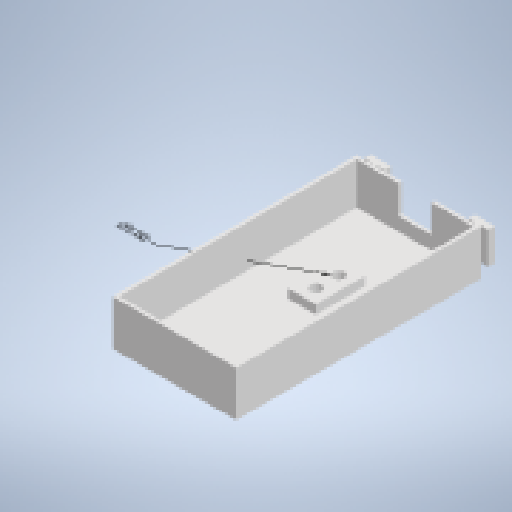
# Autodesk Inventor part: Soporte_Cuenco
Saved by Autodesk Inventor 2024 (Build 280153000, 153)
## iProperties
Created: 2024-07-17
Part Number: Soporte_Cuenco
Material: Genérico
Document SubType Name: Modeling
Designer: sergi
Density: 1 g/cm^3
Appearance: Valor por defecto
Author: sergi
Autodesk Inventor part; units mm, degrees
ref_plane "YZ Plane" through (0, 0, 0) normal (1, 0, 0) x (0, 1, 0)
ref_plane "XZ Plane" through (0, 0, 0) normal (0, 1, 0) x (-1, 0, 0)
ref_plane "XY Plane" through (0, 0, 0) normal (0, 0, 1) x (1, 0, 0)
sketch "Boceto1" plane through (0, 0, 0) normal (0, 0, 1) x (1, 0, 0)
  line L0 (-21.643, 32.4807) -> (-21.643, 43.3467) projected
  line L1 (-21.643, 43.3467) -> (-18.643, 43.3467) projected
  line L2 (-18.643, 43.3467) -> (-18.643, 34.2127) projected
  line L3 (-18.643, 34.2127) -> (-9.9759, 39.2167) projected
  line L4 (-9.9759, 39.2167) -> (9.7759, 39.2167) projected
  line L5 (9.7759, 39.2167) -> (18.443, 34.2127) projected
  line L6 (18.443, 34.2127) -> (18.443, 43.3467) projected
  line L7 (18.443, 43.3467) -> (21.443, 43.3467) projected
  line L8 (21.443, 43.3467) -> (21.443, 32.4807) projected
  line L9 (21.443, 32.4807) -> (29.5244, 27.8149) projected
  ellipse E0 centre (28.1102, 26.9984) end of major axis (26.1102, 26.9984) minor radius 1.1547 (30.1102, 26.9984) -> (29.5244, 27.8149) ccw projected
  line L10 (30.1102, 26.9984) -> (30.1102, 16.9984) projected
  line L11 (30.1102, 16.9984) -> (-30.3102, 16.9984) projected
  line L12 (-30.3102, 16.9984) -> (-30.3102, 26.9984) projected
  ellipse E1 centre (-28.3102, 26.9984) end of major axis (-30.3102, 26.9984) minor radius 1.1547 (-29.7244, 27.8149) -> (-30.3102, 26.9984) ccw projected
  line L13 (-29.7244, 27.8149) -> (-21.643, 32.4807) projected
  circle A0 centre (-50.1, -10) radius 1.5 projected
  circle A1 centre (49.9, -10) radius 1.5 projected
  circle A2 centre (49.9, 113) radius 1.5 projected
  circle A3 centre (-50.1, 113) radius 1.5 projected
  circle A4 centre (-50.1, -110) radius 1.75 projected
  circle A5 centre (49.9, -110) radius 1.75 projected
  line L14 (-22.1, 125) -> (-22.1, 110) projected
  line L15 (-22.1, 110) -> (-25.1, 110) projected
  line L16 (-25.1, 110) -> (-25.1, 125) projected
  line L17 (-25.1, 125) -> (-103.1, 125) projected
  line L18 (-103.1, 125) -> (-103.1, 100) projected
  line L19 (-103.1, 100) -> (-100.1, 100) projected
  line L20 (-100.1, 100) -> (-100.1, 75) projected
  line L21 (-100.1, 75) -> (-103.1, 75) projected
  line L22 (-103.1, 75) -> (-103.1, 50) projected
  line L23 (-103.1, 50) -> (-100.1, 50) projected
  line L24 (-100.1, 50) -> (-100.1, 25) projected
  line L25 (-100.1, 25) -> (-103.1, 25) projected
  line L26 (-103.1, 25) -> (-103.1, 0) projected
  line L27 (-103.1, 0) -> (-100.1, 0) projected
  line L28 (-100.1, 0) -> (-100.1, -25) projected
  line L29 (-100.1, -25) -> (-103.1, -25) projected
  line L30 (-103.1, -25) -> (-103.1, -50) projected
  line L31 (-103.1, -50) -> (-100.1, -50) projected
  line L32 (-100.1, -50) -> (-100.1, -75) projected
  line L33 (-100.1, -75) -> (-103.1, -75) projected
  line L34 (-103.1, -75) -> (-103.1, -100) projected
  line L35 (-103.1, -100) -> (-100.1, -100) projected
  line L36 (-100.1, -100) -> (-100.1, -125) projected
  line L37 (-100.1, -125) -> (102.9, -125) projected
  line L38 (102.9, -125) -> (102.9, -100) projected
  line L39 (102.9, -100) -> (99.9, -100) projected
  line L40 (99.9, -100) -> (99.9, -75) projected
  line L41 (99.9, -75) -> (102.9, -75) projected
  line L42 (102.9, -75) -> (102.9, -50) projected
  line L43 (102.9, -50) -> (99.9, -50) projected
  line L44 (99.9, -50) -> (99.9, -25) projected
  line L45 (99.9, -25) -> (102.9, -25) projected
  line L46 (102.9, -25) -> (102.9, 0) projected
  line L47 (102.9, 0) -> (99.9, 0) projected
  line L48 (99.9, 0) -> (99.9, 25) projected
  line L49 (99.9, 25) -> (102.9, 25) projected
  line L50 (102.9, 25) -> (102.9, 50) projected
  line L51 (102.9, 50) -> (99.9, 50) projected
  line L52 (99.9, 50) -> (99.9, 75) projected
  line L53 (99.9, 75) -> (102.9, 75) projected
  line L54 (102.9, 75) -> (102.9, 100) projected
  line L55 (102.9, 100) -> (99.9, 100) projected
  line L56 (99.9, 100) -> (99.9, 125) projected
  line L57 (99.9, 125) -> (24.9, 125) projected
  line L58 (24.9, 125) -> (24.9, 110) projected
  line L59 (24.9, 110) -> (21.9, 110) projected
  line L60 (21.9, 110) -> (21.9, 125) projected
  line L61 (24.9, 125) -> (21.9, 125)
  line L62 (22.15, 125.25) -> (22.15, 110.25)
  line L63 (22.15, 110.25) -> (24.65, 110.25)
  line L64 (24.65, 110.25) -> (24.65, 125.25)
  line L65 (24.65, 125.25) -> (100.15, 125.25)
  line L66 (100.15, 125.25) -> (100.15, 100.25)
  line L67 (100.15, 100.25) -> (103.15, 100.25)
  line L68 (103.15, 100.25) -> (103.15, 74.75)
  line L69 (103.15, 74.75) -> (100.15, 74.75)
  line L70 (100.15, 74.75) -> (100.15, 50.25)
  line L71 (100.15, 50.25) -> (103.15, 50.25)
  line L72 (103.15, 50.25) -> (103.15, 24.75)
  line L73 (103.15, 24.75) -> (100.15, 24.75)
  line L74 (100.15, 24.75) -> (100.15, 0.25)
  line L75 (100.15, 0.25) -> (103.15, 0.25)
  line L76 (103.15, 0.25) -> (103.15, -25.25)
  line L77 (103.15, -25.25) -> (100.15, -25.25)
  line L78 (100.15, -25.25) -> (100.15, -49.75)
  line L79 (100.15, -49.75) -> (103.15, -49.75)
  line L80 (103.15, -49.75) -> (103.15, -75.25)
  line L81 (103.15, -75.25) -> (100.15, -75.25)
  line L82 (100.15, -75.25) -> (100.15, -99.75)
  line L83 (100.15, -99.75) -> (103.15, -99.75)
  line L84 (103.15, -99.75) -> (103.15, -125.25)
  line L85 (103.15, -125.25) -> (-100.35, -125.25)
  line L86 (-100.35, -125.25) -> (-100.35, -100.25)
  line L87 (-100.35, -100.25) -> (-103.35, -100.25)
  line L88 (-103.35, -100.25) -> (-103.35, -74.75)
  line L89 (-103.35, -74.75) -> (-100.35, -74.75)
  line L90 (-100.35, -74.75) -> (-100.35, -50.25)
  line L91 (-100.35, -50.25) -> (-103.35, -50.25)
  line L92 (-103.35, -50.25) -> (-103.35, -24.75)
  line L93 (-103.35, -24.75) -> (-100.35, -24.75)
  line L94 (-100.35, -24.75) -> (-100.35, -0.25)
  line L95 (-100.35, -0.25) -> (-103.35, -0.25)
  line L96 (-103.35, -0.25) -> (-103.35, 25.25)
  line L97 (-103.35, 25.25) -> (-100.35, 25.25)
  line L98 (-100.35, 25.25) -> (-100.35, 49.75)
  line L99 (-100.35, 49.75) -> (-103.35, 49.75)
  line L100 (-103.35, 49.75) -> (-103.35, 75.25)
  line L101 (-103.35, 75.25) -> (-100.35, 75.25)
  line L102 (-100.35, 75.25) -> (-100.35, 99.75)
  line L103 (-100.35, 99.75) -> (-103.35, 99.75)
  line L104 (-103.35, 99.75) -> (-103.35, 125.25)
  line L105 (-103.35, 125.25) -> (-24.85, 125.25)
  line L106 (-24.85, 125.25) -> (-24.85, 110.25)
  line L107 (-24.85, 110.25) -> (-22.35, 110.25)
  line L108 (-22.35, 110.25) -> (-22.35, 125.25)
  line L109 (-22.35, 125.25) -> (22.15, 125.25)
  line L110 (24.9418, 124.75) -> (21.9418, 124.75)
  line L111 (-22.1, 125) -> (-25.1, 125)
  line L112 (-22.0582, 124.75) -> (-25.0582, 124.75)
  line L113 (7.4, 125) -> (7.4, 115) projected
  line L114 (7.4, 115) -> (-7.6, 115) projected
  line L115 (-7.6, 115) -> (-7.6, 125) projected
  line L116 (-7.6, 125) -> (-22.1, 125) projected
  line L117 (21.9, 125) -> (7.4, 125) projected
  point P0 (0, 0)
  point P1 (-22.35, 124.75)
  point P2 (-24.85, 124.75)
  point P3 (24.65, 124.75)
  point P4 (22.15, 124.75)
  dimension "d0" = 0.25
  dimension "d1" = 0.25
  dimension "d2" = 0.25
  constraints: 104 end point, 2 horizontal, 2 parallel, 48 other
  measures "d0" distance between parallel lines of L60 L62
  measures "d1" distance between parallel lines of L61 L110
  measures "d2" distance between parallel lines of L111 L112
extrude "Extrusión1" add sketch "Boceto1" against normal blind 3.5 contours L108 L107 L106 L112 | L110 L64 L63 L62
sketch "Boceto2" plane through (0, 0, -3.5) normal (0, 0, -1) x (-1, 0, 0)
  line L0 (22.35, 124.75) -> (22.35, 110.25) projected
  line L1 (22.35, 110.25) -> (24.85, 110.25) projected
  line L2 (24.85, 110.25) -> (24.85, 124.75) projected
  line L3 (24.85, 124.75) -> (22.35, 124.75) projected
  line L4 (-24.65, 124.75) -> (-24.65, 110.25) projected
  line L5 (-24.65, 110.25) -> (-22.15, 110.25) projected
  line L6 (-22.15, 110.25) -> (-22.15, 124.75) projected
  line L7 (-22.15, 124.75) -> (-24.65, 124.75) projected
  circle A0 centre (50.1, -10) radius 1.5 projected
  circle A1 centre (-49.9, -10) radius 1.5 projected
  circle A2 centre (-49.9, 113) radius 1.5 projected
  circle A3 centre (50.1, 113) radius 1.5 projected
  circle A4 centre (50.1, -110) radius 1.75 projected
  circle A5 centre (-49.9, -110) radius 1.75 projected
  line L8 (25.1, 125) -> (25.1, 110) projected
  line L9 (25.1, 110) -> (22.1, 110) projected
  line L10 (22.1, 110) -> (22.1, 125) projected
  line L11 (22.1, 125) -> (7.6, 125) projected
  line L12 (-21.9, 125) -> (-21.9, 110) projected
  line L13 (-21.9, 110) -> (-24.9, 110) projected
  line L14 (-24.9, 110) -> (-24.9, 125) projected
  line L15 (-24.9, 125) -> (-99.9, 125) projected
  line L16 (-99.9, 125) -> (-99.9, 100) projected
  line L17 (-99.9, 100) -> (-102.9, 100) projected
  line L18 (-102.9, 100) -> (-102.9, 75) projected
  line L19 (-102.9, 75) -> (-99.9, 75) projected
  line L20 (-99.9, 75) -> (-99.9, 50) projected
  line L21 (-99.9, 50) -> (-102.9, 50) projected
  line L22 (-102.9, 50) -> (-102.9, 25) projected
  line L23 (-102.9, 25) -> (-99.9, 25) projected
  line L24 (-99.9, 25) -> (-99.9, 0) projected
  line L25 (-99.9, 0) -> (-102.9, 0) projected
  line L26 (-102.9, 0) -> (-102.9, -25) projected
  line L27 (-102.9, -25) -> (-99.9, -25) projected
  line L28 (-99.9, -25) -> (-99.9, -50) projected
  line L29 (-99.9, -50) -> (-102.9, -50) projected
  line L30 (-102.9, -50) -> (-102.9, -75) projected
  line L31 (-102.9, -75) -> (-99.9, -75) projected
  line L32 (-99.9, -75) -> (-99.9, -100) projected
  line L33 (-99.9, -100) -> (-102.9, -100) projected
  line L34 (-102.9, -100) -> (-102.9, -125) projected
  line L35 (-102.9, -125) -> (100.1, -125) projected
  line L36 (100.1, -125) -> (100.1, -100) projected
  line L37 (100.1, -100) -> (103.1, -100) projected
  line L38 (103.1, -100) -> (103.1, -75) projected
  line L39 (103.1, -75) -> (100.1, -75) projected
  line L40 (100.1, -75) -> (100.1, -50) projected
  line L41 (100.1, -50) -> (103.1, -50) projected
  line L42 (103.1, -50) -> (103.1, -25) projected
  line L43 (103.1, -25) -> (100.1, -25) projected
  line L44 (100.1, -25) -> (100.1, 0) projected
  line L45 (100.1, 0) -> (103.1, 0) projected
  line L46 (103.1, 0) -> (103.1, 25) projected
  line L47 (103.1, 25) -> (100.1, 25) projected
  line L48 (100.1, 25) -> (100.1, 50) projected
  line L49 (100.1, 50) -> (103.1, 50) projected
  line L50 (103.1, 50) -> (103.1, 75) projected
  line L51 (103.1, 75) -> (100.1, 75) projected
  line L52 (100.1, 75) -> (100.1, 100) projected
  line L53 (100.1, 100) -> (103.1, 100) projected
  line L54 (103.1, 100) -> (103.1, 125) projected
  line L55 (21.643, 43.3467) -> (21.643, 32.4807) projected
  line L56 (21.643, 32.4807) -> (29.7244, 27.8149) projected
  ellipse E0 centre (28.3102, 26.9984) end of major axis (30.3102, 26.9984) minor radius 1.1547 (30.3102, 26.9984) -> (29.7244, 27.8149) ccw projected
  line L57 (30.3102, 26.9984) -> (30.3102, 16.9984) projected
  line L58 (30.3102, 16.9984) -> (-30.1102, 16.9984) projected
  line L59 (-30.1102, 16.9984) -> (-30.1102, 26.9984) projected
  ellipse E1 centre (-28.1102, 26.9984) end of major axis (-26.1102, 26.9984) minor radius 1.1547 (-29.5244, 27.8149) -> (-30.1102, 26.9984) ccw projected
  line L60 (-29.5244, 27.8149) -> (-21.443, 32.4807) projected
  line L61 (-21.443, 32.4807) -> (-21.443, 43.3467) projected
  line L62 (-21.443, 43.3467) -> (-18.443, 43.3467) projected
  line L63 (-18.443, 43.3467) -> (-18.443, 34.2127) projected
  line L64 (-18.443, 34.2127) -> (-9.7759, 39.2167) projected
  line L65 (-9.7759, 39.2167) -> (9.9759, 39.2167) projected
  line L66 (9.9759, 39.2167) -> (18.643, 34.2127) projected
  line L67 (18.643, 34.2127) -> (18.643, 43.3467) projected
  line L68 (18.643, 43.3467) -> (21.643, 43.3467) projected
  line L69 (22.1, 125) -> (19.1, 125)
  line L70 (19.1, 125) -> (28.1, 125)
  line L71 (28.1, 125) -> (28.1, 110.25)
  line L72 (28.1, 110.25) -> (19.1, 110.25)
  line L73 (19.1, 110.25) -> (19.1, 125)
  line L74 (-25, 125) -> (-28, 125)
  line L75 (-28, 125) -> (-19, 125)
  line L76 (-19, 125) -> (-19, 110.25)
  line L77 (-19, 110.25) -> (-28, 110.25)
  line L78 (-28, 110.25) -> (-28, 125)
  line L79 (-28, 124.75) -> (28.1, 124.75)
  line L80 (7.6, 125) -> (7.6, 115) projected
  line L81 (7.6, 115) -> (-7.4, 115) projected
  line L82 (-7.4, 115) -> (-7.4, 125) projected
  line L83 (-7.4, 125) -> (-21.9, 125) projected
  line L84 (103.1, 125) -> (25.1, 125) projected
  point P0 (0, 0)
  point P1 (-19, 124.75)
  point P2 (19.1, 124.75)
  point P3 (100, 125)
  point P4 (-24.65, 124.75)
  point P5 (-22.15, 124.75)
  point P6 (24.85, 124.75)
  point P7 (22.35, 124.75)
  point P8 (22.35, 110.25)
  point P9 (24.85, 110.25)
  point P10 (25.1, 110.25)
  point P11 (22.1, 110.25)
  point P12 (28.0918, 124.9919)
  point P13 (25.1, 125)
  point P14 (25.1, 125)
  dimension "d5" = 3
  dimension "d6" = 3
  dimension "d7" = 3
  constraints: 22 end point, 4 parallel, 3 perpendicular, 3 point on line, 2 horizontal, 2 other
  measures "d5" distance of L10.end L69.end
  measures "d6" distance between parallel lines of L71 L8
  measures "d7" distance of L74.start L75.start
extrude "Extrusión2" add sketch "Boceto2" along normal blind 3 contours L3 L2 L1 L0 | L0 L72 L10 L79 | L79 L8 L72 L2 | L10 L72 L73 L79 | L79 L71 L72 L8 | L76 L77 L12 L79 | L12 L77 L6 L79 | L6 L5 L4 L7 | L4 L77 L14 L79 | L14 L77 L78 L79
ref_plane "Plano de trabajo1" through (-6.45, 111.85, 105.625) normal (0, 0, 1) x (1, 0, 0)
sketch "Boceto3" plane through (0, 0, 0) normal (0, 0, 1) x (1, 0, 0)
  line L0 (-28.1, 124.75) -> (-19.1, 124.75) projected
  line L1 (-19.1, 124.75) -> (-19.1, 110.25) projected
  line L2 (-19.1, 110.25) -> (-28.1, 110.25) projected
  line L3 (-28.1, 110.25) -> (-28.1, 124.75) projected
  line L4 (19, 124.75) -> (28, 124.75) projected
  line L5 (28, 124.75) -> (28, 110.25) projected
  line L6 (28, 110.25) -> (19, 110.25) projected
  line L7 (19, 110.25) -> (19, 124.75) projected
  line L8 (28, 110.25) -> (-28.1, 110.25)
  line L9 (-28.1, 110.25) -> (-28.1, 124.75)
  line L10 (-28.1, 124.75) -> (28, 124.75)
  line L11 (28, 124.75) -> (28, 110.25)
  line L12 (28, 124.75) -> (-28.1, 124.75)
  line L13 (-28.1, 124.75) -> (-28.1, 104.75)
  line L14 (-28.1, 104.75) -> (28, 104.75)
  line L15 (28, 104.75) -> (28, 124.75)
  dimension "d25" = 20
  constraints: 16 end point, 4 parallel, 2 horizontal, 2 perpendicular
  measures "d25" distance of L13.end L12.end
extrude "Extrusión3" add sketch "Boceto3" along normal blind 110.625
shell "Vaciado1" thickness 1.6 removed faces 1 at (7.35, 124.75, 73.75)
sketch "Boceto7" plane through (19, 110.25, -6.5) normal (0, -1, 0) x (1, 0, 0)
  circle A0 centre (-19.1, 106.5) radius 6.4 projected
  circle A1 centre (-19.1, 106.5) radius 9
  line L0 (-10.1, 106.5) -> (1.4, 106.5) construction
  line L1 (-10.1, 106.5) -> (-28.1, 106.5)
  line L2 (-28.1, 106.5) -> (-28.1, 123.2114)
  line L3 (-28.1, 123.2114) -> (-10.1, 123.2114)
  line L4 (-10.1, 123.2114) -> (-10.1, 106.5)
  point P0 (-19, 6.5)
  dimension "d20" = 18
  dimension "d24" = 18
  constraints: 10 end point, 2 horizontal, 2 parallel, 1 coincident, 1 perpendicular, 3 other
  measures "d24" distance of L2.end L3.end
extrude "Extrusión7" cut sketch "Boceto7" along normal blind 10 contours L1 A0 | L1 A1 A0 | A0 L1 A1 | A0 L1
sketch "Boceto6" plane through (24.65, 124.75, -3.5) normal (0, 1, 0) x (1, 0, 0)
  line L0 (0, -3.5) -> (-49.5, -3.5)
  line L1 (1.75, -5.1) -> (1.75, -112.525) projected
  line L2 (3.35, -3.5) -> (3.35, -114.125) projected
  line L3 (3.35, -3.5) -> (0, -3.5) projected
  line L4 (0, -3.5) -> (0, 0) projected
  line L5 (0, 0) -> (3.35, 0) projected
  line L6 (3.35, 0) -> (3.35, 3) projected
  line L7 (-5.65, 3) -> (3.35, 3) projected
  line L8 (-5.65, 0) -> (-5.65, 3) projected
  line L9 (-5.65, 0) -> (-2.5, 0) projected
  line L10 (-2.5, -3.5) -> (-2.5, 0) projected
  line L11 (-2.5, -3.5) -> (-47, -3.5) projected
  line L12 (-47, -3.5) -> (-47, 0) projected
  line L13 (-47, 0) -> (-43.75, 0) projected
  line L14 (-43.75, 0) -> (-43.75, 3) projected
  line L15 (-52.75, 3) -> (-43.75, 3) projected
  line L16 (-52.75, 0) -> (-52.75, 3) projected
  line L17 (-52.75, 0) -> (-49.5, 0) projected
  line L18 (-49.5, -3.5) -> (-49.5, 0) projected
  line L19 (-49.5, -3.5) -> (-52.75, -3.5) projected
  line L20 (-52.75, -3.5) -> (-52.75, -114.125) projected
  line L21 (-51.15, -112.525) -> (-51.15, -5.1) projected
  line L22 (-51.15, -5.1) -> (1.75, -5.1) projected
  line L23 (1.75, -112.525) -> (-51.15, -112.525) projected
  line L24 (3.35, -114.125) -> (-52.75, -114.125) projected
  point P0 (-24.65, -3.5)
  constraints: 2 end point
extrude "Extrusión6" add sketch "Boceto6" along normal blind 3 contours L3 L2 L24 L20 L19 L0
sketch "Boceto8" plane through (-26.5, 106.35, 1.6) normal (0, 0, 1) x (1, 0, 0)
  line L0 (33.9, 8.65) -> (18.9, 8.65) projected
  line L1 (33.9, 18.65) -> (33.9, 8.65) projected
  line L2 (18.9, 18.65) -> (18.9, 8.65) projected
  line L3 (54.5, 21.4) -> (-1.6, 21.4) projected
  line L4 (33.9, 8.65) -> (18.9, 8.65)
  line L5 (18.9, 8.65) -> (18.9, 21.4)
  line L6 (18.9, 21.4) -> (33.9, 21.4)
  line L7 (33.9, 21.4) -> (33.9, 8.65)
  point P0 (26.5, -106.35)
  constraints: 8 end point, 2 parallel, 1 horizontal, 1 perpendicular, 1 point on line
extrude "Extrusión8" cut sketch "Boceto8" against normal blind 3
sketch "Boceto9" plane through (-26.5, 106.35, 1.6) normal (0, 1, 0) x (1, 0, 0)
  circle A0 centre (26.45, -34.65) radius 2 projected
  circle A1 centre (26.45, -44.85) radius 2 projected
  circle A2 centre (26.4, -98.4) radius 2 projected
  circle A3 centre (26.4, -88.2) radius 2 projected
  line L0 (20.05, -29.025) -> (20.05, -104.025) projected
  line L1 (20.05, -104.025) -> (32.75, -104.025) projected
  line L2 (32.75, -29.025) -> (32.75, -104.025) projected
  line L3 (20.05, -29.025) -> (32.75, -29.025) projected
  circle A4 centre (26.45, -44.85) radius 6.4
  circle A5 centre (26.45, -34.65) radius 6.4
  line L4 (32.75, -51.25) -> (20.05, -51.25)
  line L5 (20.05, -51.25) -> (20.05, -28.25)
  line L6 (20.05, -28.25) -> (32.75, -28.25)
  line L7 (32.75, -28.25) -> (32.75, -51.25)
  circle A6 centre (26.45, -34.65) radius 2.8
  circle A7 centre (26.45, -44.85) radius 2.8
  point P0 (26.5, 1.6)
  dimension "d30" = 5.6
  dimension "d31" = 5.6
  constraints: 8 end point, 4 centre point, 4 coincident, 2 parallel, 2 point on line, 2 tangent, 1 horizontal, 1 perpendicular
  measures "d30" diameter of A6
  measures "d31" diameter of A7
extrude "Extrusión9" add sketch "Boceto9" along normal blind 4 contours L0 A4 L4 | L0 A5 A4 | A4 A5 L2 | A4 L2 L4 | L0 L3 A5 | A5 L3 L2 A4 | A4 A5 | A5 L2 A4 | L3 L2 A5
